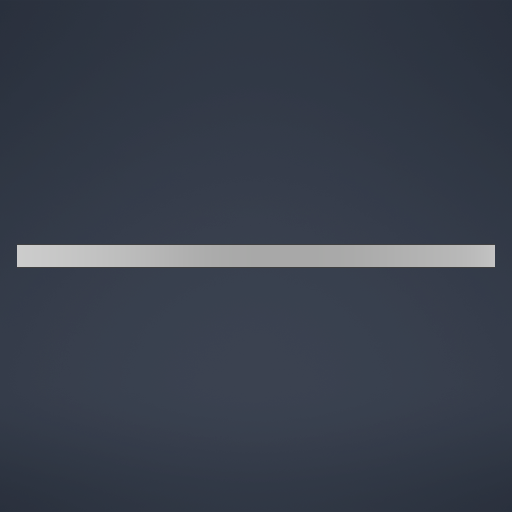
# Autodesk Inventor part: 260mm Housing 1
Saved by Autodesk Inventor 2025 (Build 290162000, 162)
## iProperties
Created: 2024-10-30
Part Number: 260mm Housing 1
Material: Generic
Document SubType Name: Modeling
Designer: mayhe
Density: 1 g/cm^3
Appearance: Default
Author: mayhe
Autodesk Inventor part; units mm, degrees
ref_plane "YZ Plane" through (0, 0, 0) normal (1, 0, 0) x (0, 1, 0)
ref_plane "XZ Plane" through (0, 0, 0) normal (0, 1, 0) x (-1, 0, 0)
ref_plane "XY Plane" through (0, 0, 0) normal (0, 0, 1) x (1, 0, 0)
sketch "Sketch1" plane through (0, 0, 0) normal (0, 1, 0) x (-1, 0, 0)
  circle A0 centre (0, 0) radius 150
  circle A1 centre (0, 0) radius 100
  circle A2 centre (0, 0) radius 120.625
  circle A3 centre (0, 0) radius 140
  circle A4 centre (-140, 0) radius 2.75
  line L0 (-144.375, 2.5259) -> (-140, 5.0518)
  line L1 (-140, 5.0518) -> (-135.625, 2.5259)
  line L2 (-135.625, 2.5259) -> (-135.625, -2.5259)
  line L3 (-135.625, -2.5259) -> (-140, -5.0518)
  line L4 (-140, -5.0518) -> (-144.375, -2.5259)
  line L5 (-144.375, -2.5259) -> (-144.375, 2.5259)
  circle A5 centre (-113.2624, -82.2899) radius 2.75
  line L6 (-118.2865, -82.818) -> (-116.2318, -78.2029)
  line L7 (-116.2318, -78.2029) -> (-111.2076, -77.6749)
  line L8 (-111.2076, -77.6749) -> (-108.2382, -81.7619)
  line L9 (-108.2382, -81.7619) -> (-110.293, -86.3769)
  line L10 (-110.293, -86.3769) -> (-115.3171, -86.905)
  line L11 (-115.3171, -86.905) -> (-118.2865, -82.818)
  circle A6 centre (-43.2624, -133.1479) radius 2.75
  line L12 (-47.0166, -136.5282) -> (-48.0669, -131.5868)
  line L13 (-48.0669, -131.5868) -> (-44.3127, -128.2065)
  line L14 (-44.3127, -128.2065) -> (-39.5081, -129.7676)
  line L15 (-39.5081, -129.7676) -> (-38.4578, -134.709)
  line L16 (-38.4578, -134.709) -> (-42.212, -138.0893)
  line L17 (-42.212, -138.0893) -> (-47.0166, -136.5282)
  circle A7 centre (43.2624, -133.1479) radius 2.75
  line L18 (42.212, -138.0893) -> (38.4578, -134.709)
  line L19 (38.4578, -134.709) -> (39.5081, -129.7676)
  line L20 (39.5081, -129.7676) -> (44.3127, -128.2065)
  line L21 (44.3127, -128.2065) -> (48.0669, -131.5868)
  line L22 (48.0669, -131.5868) -> (47.0166, -136.5282)
  line L23 (47.0166, -136.5282) -> (42.212, -138.0893)
  circle A8 centre (113.2624, -82.2899) radius 2.75
  line L24 (115.3171, -86.905) -> (110.293, -86.3769)
  line L25 (110.293, -86.3769) -> (108.2382, -81.7619)
  line L26 (108.2382, -81.7619) -> (111.2076, -77.6749)
  line L27 (111.2076, -77.6749) -> (116.2318, -78.2029)
  line L28 (116.2318, -78.2029) -> (118.2865, -82.818)
  line L29 (118.2865, -82.818) -> (115.3171, -86.905)
  circle A9 centre (140, 0) radius 2.75
  line L30 (144.375, -2.5259) -> (140, -5.0518)
  line L31 (140, -5.0518) -> (135.625, -2.5259)
  line L32 (135.625, -2.5259) -> (135.625, 2.5259)
  line L33 (135.625, 2.5259) -> (140, 5.0518)
  line L34 (140, 5.0518) -> (144.375, 2.5259)
  line L35 (144.375, 2.5259) -> (144.375, -2.5259)
  circle A10 centre (113.2624, 82.2899) radius 2.75
  line L36 (118.2865, 82.818) -> (116.2318, 78.2029)
  line L37 (116.2318, 78.2029) -> (111.2076, 77.6749)
  line L38 (111.2076, 77.6749) -> (108.2382, 81.7619)
  line L39 (108.2382, 81.7619) -> (110.293, 86.3769)
  line L40 (110.293, 86.3769) -> (115.3171, 86.905)
  line L41 (115.3171, 86.905) -> (118.2865, 82.818)
  circle A11 centre (43.2624, 133.1479) radius 2.75
  line L42 (47.0166, 136.5282) -> (48.0669, 131.5868)
  line L43 (48.0669, 131.5868) -> (44.3127, 128.2065)
  line L44 (44.3127, 128.2065) -> (39.5081, 129.7676)
  line L45 (39.5081, 129.7676) -> (38.4578, 134.709)
  line L46 (38.4578, 134.709) -> (42.212, 138.0893)
  line L47 (42.212, 138.0893) -> (47.0166, 136.5282)
  circle A12 centre (-43.2624, 133.1479) radius 2.75
  line L48 (-42.212, 138.0893) -> (-38.4578, 134.709)
  line L49 (-38.4578, 134.709) -> (-39.5081, 129.7676)
  line L50 (-39.5081, 129.7676) -> (-44.3127, 128.2065)
  line L51 (-44.3127, 128.2065) -> (-48.0669, 131.5868)
  line L52 (-48.0669, 131.5868) -> (-47.0166, 136.5282)
  line L53 (-47.0166, 136.5282) -> (-42.212, 138.0893)
  circle A13 centre (-113.2624, 82.2899) radius 2.75
  line L54 (-115.3171, 86.905) -> (-110.293, 86.3769)
  line L55 (-110.293, 86.3769) -> (-108.2382, 81.7619)
  line L56 (-108.2382, 81.7619) -> (-111.2076, 77.6749)
  line L57 (-111.2076, 77.6749) -> (-116.2318, 78.2029)
  line L58 (-116.2318, 78.2029) -> (-118.2865, 82.818)
  line L59 (-118.2865, 82.818) -> (-115.3171, 86.905)
  point P0 (-144.375, 0)
  point P1 (-116.8018, -84.8615)
  point P2 (-44.6143, -137.3088)
  point P3 (44.6143, -137.3088)
  point P4 (116.8018, -84.8615)
  point P5 (144.375, 0)
  point P6 (116.8018, 84.8615)
  point P7 (44.6143, 137.3088)
  point P8 (-44.6143, 137.3088)
  point P9 (-116.8018, 84.8615)
  dimension "d20" = 280
  dimension "d0" = 300
  dimension "d1" = 200
  dimension "d19" = 241.25
  dimension "d21" = 5.5
  dimension "d25" = 360
  dimension "d52" = 8.75
  constraints: 120 end point, 13 centre point, 7 coincident, 1 horizontal alignment, 1 midpoint, 176 other
  measures "d0" diameter of A0
  measures "d1" diameter of A1
  measures "d19" diameter of A2
  measures "d21" diameter of A4
  measures "d52" distance between parallel lines of L2 L5
extrude "Extrusion1" add sketch "Sketch1" along normal blind 2 contours A0 | A2 | L33 L32 L31 A3 L27 L26 L25 L21 L20 L19 L15 L14 L13 L9 L8 L7 L3 L2 L1 L57 L56 L55 L51 L50 L49 L45 L44 L43 L39 L38 L37
extrude "Extrusion3" add sketch "Sketch1" along normal blind 4.25 contours A0 | A2 | L33 L32 L31 A3 L27 L26 L25 L21 L20 L19 L15 L14 L13 L9 L8 L7 L3 L2 L1 L57 L56 L55 L51 L50 L49 L45 L44 L43 L39 L38 L37
sketch "Sketch4" plane through (0, 4.25, 0) normal (0, 1, 0) x (1, 0, 0)
  circle A0 centre (0, 0) radius 100
  circle A1 centre (0, 0) radius 150
  circle A2 centre (-140, 0) radius 2.75
  circle A3 centre (0, 0) radius 140
  circle A4 centre (-113.2624, -82.2899) radius 2.75
  circle A5 centre (-43.2624, -133.1479) radius 2.75
  circle A6 centre (43.2624, -133.1479) radius 2.75
  circle A7 centre (113.2624, -82.2899) radius 2.75
  circle A8 centre (140, 0) radius 2.75
  circle A9 centre (113.2624, 82.2899) radius 2.75
  circle A10 centre (43.2624, 133.1479) radius 2.75
  circle A11 centre (-43.2624, 133.1479) radius 2.75
  circle A12 centre (-113.2624, 82.2899) radius 2.75
  dimension "d55" = 200
  dimension "d58" = 360
  constraints: 12 centre point, 4 coincident, 1 horizontal alignment, 23 other
  measures "d55" diameter of A0
extrude "Extrusion4" add sketch "Sketch4" along normal blind 10.75 contours A1 | A2 A3 A12 A11 A10 A9 A8 A7 A6 A5 A4
sketch "Sketch3" plane through (0, 15, 0) normal (0, 1, 0) x (1, 0, 0)
  circle A0 centre (0, 0) radius 125
  circle A1 centre (0, 125) radius 2.75
  circle A2 centre (-73.4732, 101.1271) radius 2.75
  circle A3 centre (-118.8821, 38.6271) radius 2.75
  circle A4 centre (-118.8821, -38.6271) radius 2.75
  circle A5 centre (-73.4732, -101.1271) radius 2.75
  circle A6 centre (0, -125) radius 2.75
  circle A7 centre (73.4732, -101.1271) radius 2.75
  circle A8 centre (118.8821, -38.6271) radius 2.75
  circle A9 centre (118.8821, 38.6271) radius 2.75
  circle A10 centre (73.4732, 101.1271) radius 2.75
  circle A11 centre (0, 0) radius 120.625
  dimension "d13" = 250
  dimension "d14" = 5.5
  dimension "d17" = 360
  dimension "d35" = 241.25
  constraints: 11 centre point, 2 coincident, 1 vertical alignment, 23 other
  measures "d14" diameter of A1
  measures "d35" diameter of A11
extrude "Extrusion5" cut sketch "Sketch3" against normal blind 2.125 contours A11
hole "Hole1" at (-118.8821, 15, 38.6271) at (-73.4732, 15, 101.1271) at (0, 15, 125) at (73.4732, 15, 101.1271) at (118.8821, 15, 38.6271) at (118.8821, 15, -38.6271) at (73.4732, 15, -101.1271) at (0, 15, -125) at (-73.4732, 15, -101.1271) at (-118.8821, 15, -38.6271) direction (0, -1, 0) diameter 5.5 end through all counterbore diameter 10.475 counterbore depth 7.375
sketch "Sketch5" plane through (0, 0, 0) normal (1, 0, 0) x (0, 1, 0)
  line L0 (12.875, 120.5918) -> (12.875, 99.2233) projected
  line L1 (0, -150) -> (0, 150) projected
  line L2 (14.875, 112.5) -> (10.875, 112.5)
  line L3 (10.875, 112.5) -> (10.875, 116.5)
  line L4 (10.875, 116.5) -> (14.875, 116.5)
  line L5 (14.875, 116.5) -> (14.875, 112.5)
  line L6 (14.875, 112.5) -> (10.875, 116.5) construction
  line L7 (10.875, 112.5) -> (14.875, 116.5) construction
  line L8 (12.875, 100) -> (0, 100) projected
  line L9 (12.875, 100) -> (0, 100)
  line L10 (2, 116.5) -> (-2, 116.5)
  line L11 (-2, 116.5) -> (-2, 112.5)
  line L12 (-2, 112.5) -> (2, 112.5)
  line L13 (2, 112.5) -> (2, 116.5)
  line L14 (2, 116.5) -> (-2, 112.5) construction
  line L15 (-2, 116.5) -> (2, 112.5) construction
  line L16 (-5.375, 0) -> (18.25, 0) projected
  point P0 (0, 0)
  point P1 (12.875, 114.5)
  point P2 (0, 114.5)
  dimension "d45" = 4
  dimension "d46" = 4
  dimension "d48" = 14.5
  dimension "d49" = 4
  dimension "d50" = 4
  constraints: 26 end point, 5 point on line, 4 midpoint, 4 parallel, 2 horizontal, 2 perpendicular, 2 vertical alignment
  measures "d45" distance of L3.end L4.end
  measures "d46" distance of L2.end L3.end
  measures "d48" distance from line of L8 point (12.875, 114.5)
  measures "d49" distance of L12.end L11.end
  measures "d50" distance of L11.end L10.end
revolve "Revolution1" cut sketch "Sketch5" angle 360 about axis through (0, -10, 0) along (0, 1, 0)
extrude "Extrusion6" cut sketch "Sketch1" along normal blind 5.65 contours A3 A9 | A3 A9 | A9 A3 L31 L32 L33 | A3 L33 L34 L35 L30 L31 A9 | L37 L38 L39 A3 A10 | A3 A10 L39 L40 L41 L36 L37 | L27 L28 L29 L24 L25 A3 A8 | A3 A8 L25 L26 L27 | A10 A3 | A3 A10 | A8 A3 | A3 A8 | L43 L44 L45 A3 A11 | A3 A11 L45 L46 L47 L42 L43 | L21 L22 L23 L18 L19 A3 A7 | A3 A7 L19 L20 L21 | A11 A3 | A3 A11 | A7 A3 | A3 A7 | L49 L50 L51 A3 A12 | A3 A12 L51 L52 L53 L48 L49 | L15 L16 L17 L12 L13 A3 A6 | A3 A6 L13 L14 L15 | A12 A3 | A3 A12 | A6 A3 | A3 A6 | L55 L56 L57 A3 A13 | A3 A13 L57 L58 L59 L54 L55 | L9 L10 L11 L6 L7 A3 A5 | A3 A5 L7 L8 L9 | A13 A3 | A3 A13 | A5 A3 | A3 A5 | L1 L2 L3 A3 A4 | A3 A4 L3 L4 L5 L0 L1 | A4 A3 | A3 A4
body "Solid1"
